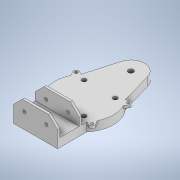
# Autodesk Inventor part: GripperBase
Saved by Autodesk Inventor 2020 (Build 240168000, 168)
## iProperties
Created: 2019-11-04
Part Number: GripperBase
Material: Generic
Document SubType Name: Modeling
Designer: kaspe
Density: 1 g/cm^3
Appearance: Default
Author: kaspe
Autodesk Inventor part; units mm, degrees
ref_plane "YZ Plane" through (0, 0, 0) normal (1, 0, 0) x (0, 1, 0)
ref_plane "XZ Plane" through (0, 0, 0) normal (0, 1, 0) x (-1, 0, 0)
ref_plane "XY Plane" through (0, 0, 0) normal (0, 0, 1) x (1, 0, 0)
sketch "Sketch1" plane through (0, 0, 0) normal (0, 1, 0) x (-1, 0, 0)
  circle A0 centre (0, 0) radius 31.65
  circle A1 centre (0, 0) radius 33.15
  dimension "d0" = 63.3
  dimension "d1" = 66.3
  constraints: 2 centre point, 2 coincident
  measures "d0" diameter of A0
  measures "d1" diameter of A1
extrude "Extrusion1" add sketch "Sketch1" along normal blind 9.8 contours A0 | A1
sketch "Sketch2" plane through (0, 0, 0) normal (0, -1, 0) x (1, 0, 0)
  circle A0 centre (0, 0) radius 31.65
  dimension "d4" = 63.3
  constraints: 1 centre point, 1 coincident
  measures "d4" diameter of A0
extrude "Extrusion2" cut sketch "Sketch2" against normal blind 6.5
sketch "Sketch3" plane through (0, 9.8, 0) normal (0, 1, 0) x (1, 0, 0)
  circle A0 centre (0, 0) radius 25
  line L0 (0, 0) -> (17.6777, 17.6777)
  line L1 (0, 0) -> (25, 0) construction
  line L2 (0, 0) -> (-17.6777, 17.6777)
  line L3 (0, 0) -> (-17.6777, -17.6777)
  line L4 (0, 0) -> (17.6777, -17.6777)
  circle A1 centre (-17.6777, 17.6777) radius 2.55
  circle A2 centre (17.6777, 17.6777) radius 2.55
  circle A3 centre (17.6777, -17.6777) radius 2.55
  circle A4 centre (-17.6777, -17.6777) radius 2.55
  circle A5 centre (0, 25) radius 3.05
  dimension "d7" = 50
  dimension "d8" = 45
  dimension "d9" = 5.1
  dimension "d10" = 5.1
  dimension "d11" = 5.1
  dimension "d12" = 5.1
  dimension "d13" = 6.1
  constraints: 10 end point, 6 centre point, 6 point on circle, 4 coincident, 1 equal length, 1 horizontal, 1 perpendicular, 1 point on line
  measures "d7" diameter of A0
  measures "d8" angle of L1 L0
  measures "d9" diameter of A1
  measures "d10" diameter of A2
  measures "d11" diameter of A3
  measures "d12" diameter of A4
  measures "d13" diameter of A5
extrude "Extrusion3" cut sketch "Sketch3" against normal blind 6.5 contours A2 L0 A0 | A0 A2 | A3 A0 | A0 L4 A3 | L0 A2 A0 | A0 A3 L4 | A5 A0 | A0 A5 | A1 A0 L2 | L2 A0 A1 | A4 A0 L3 | L3 A0 A4 | A4 A0 | A0 A1
sketch "Sketch4" plane through (0, 9.8, 0) normal (0, 1, 0) x (1, 0, 0)
  circle A0 centre (0, 0) radius 33.15 projected
  line L0 (0, 33.15) -> (0, -33.15)
  constraints: 2 end point, 2 point on circle, 1 vertical
ref_plane "Work Plane1" through (0, 9.8, 33.15) normal (0, 0, 1) x (1, 0, 0)
ref_plane "Work Plane2" through (0, 9.8, -33.15) normal (0, 0, -1) x (-1, 0, 0)
sketch "Sketch5" plane through (0, 9.8, -33.15) normal (0, 0, -1) x (-1, 0, 0)
  line L0 (33.15, 0) -> (-33.15, 0) projected
  line L1 (0, 0) -> (25, 0)
  line L2 (0, 0) -> (-25, 0)
  line L3 (33.15, -9.8) -> (-33.15, -9.8) projected
  line L4 (-25, 0) -> (25, 0)
  line L5 (25, 0) -> (25, -9.8)
  line L6 (25, -9.8) -> (-25, -9.8)
  line L7 (-25, -9.8) -> (-25, 0)
  point P0 (0, -9.8)
  dimension "d16" = 25
  dimension "d17" = 25
  constraints: 12 end point, 3 point on line, 2 parallel, 1 horizontal, 1 midpoint, 1 perpendicular
  measures "d16" distance of L1.start L1.end
  measures "d17" distance of L1.start L2.end
extrude "Extrusion4" add sketch "Sketch5" against normal blind 11.75
sketch "Sketch6" plane through (0, 9.8, 33.15) normal (0, 0, 1) x (1, 0, 0)
  line L0 (-25, 0) -> (25, 0) projected
  line L1 (0, 0) -> (-25, 0)
  line L2 (-25, 0) -> (-25, -9.8) projected
  line L3 (25, -9.8) -> (25, 0) projected
  line L4 (-25, 0) -> (25, 0)
  line L5 (25, 0) -> (25, -9.8)
  line L6 (25, -9.8) -> (-25, -9.8)
  line L7 (-25, -9.8) -> (-25, 0)
  point P0 (0, -9.8)
  dimension "d20" = 25
  dimension "d21" = 50
  constraints: 10 end point, 2 parallel, 1 collinear, 1 horizontal, 1 midpoint, 1 perpendicular
  measures "d20" distance of L1.start L0.start
  measures "d21" distance of L3.start L6.end
extrude "Extrusion5" add sketch "Sketch6" against normal blind 12.25
sketch "Sketch8" plane through (0, 9.8, 33.15) normal (0, 0, 1) x (1, 0, 0)
  line L0 (-25, -9.8) -> (25, -9.8) projected
  line L1 (25, 0) -> (25, -9.8) projected
  line L2 (-25, -9.8) -> (25, -9.8)
  line L3 (25, -9.8) -> (25, 0)
  line L4 (25, 0) -> (-25, 0)
  line L5 (-25, 0) -> (-25, -9.8)
  point P0 (0, -9.8)
  constraints: 8 end point, 2 parallel, 1 horizontal, 1 perpendicular
extrude "Extrusion6" add sketch "Sketch8" along normal blind 22
sketch "Sketch9" plane through (0, 9.8, 0) normal (0, 1, 0) x (1, 0, 0)
  line L0 (-25, -55.15) -> (-25, -21.7698) projected
  line L1 (25, -21.7698) -> (25, -55.15) projected
  line L2 (-25, -55.15) -> (25, -55.15)
  line L3 (25, -55.15) -> (25, -52.65)
  line L4 (25, -52.65) -> (-25, -52.65)
  line L5 (-25, -52.65) -> (-25, -55.15)
  point P0 (0, 0)
  dimension "d26" = 2.5
  constraints: 8 end point, 2 parallel, 1 horizontal, 1 perpendicular, 1 point on line
  measures "d26" distance of L3.end L2.end
extrude "Extrusion7" add sketch "Sketch9" along normal blind 19
sketch "Sketch11" plane through (0, 9.8, 0) normal (0, 1, 0) x (1, 0, 0)
  line L0 (25, -21.7698) -> (25, -52.65) projected
  line L1 (-25, -52.65) -> (-25, -21.7698) projected
  line L2 (25, -52.65) -> (-25, -52.65)
  line L3 (-25, -52.65) -> (-25, -30.55)
  line L4 (-25, -30.55) -> (25, -30.55)
  line L5 (25, -30.55) -> (25, -52.65)
  line L6 (25, -30.55) -> (-25, -30.55)
  line L7 (-25, -30.55) -> (-25, -28.05)
  line L8 (-25, -28.05) -> (25, -28.05)
  line L9 (25, -28.05) -> (25, -30.55)
  point P0 (0, 0)
  dimension "d39" = 22.1
  dimension "d40" = 2.5
  constraints: 16 end point, 4 parallel, 2 horizontal, 2 perpendicular, 2 point on line
  measures "d39" distance of L2.end L3.end
  measures "d40" distance of L6.end L7.end
extrude "Extrusion9" add sketch "Sketch11" along normal blind 19 contours L0 L4 L1 L8
sketch "Sketch10" plane through (0, 9.8, 55.15) normal (0, 0, 1) x (1, 0, 0)
  line L0 (-25, 0) -> (25, 0) projected
  line L1 (25, -9.8) -> (25, 19) projected
  line L2 (-25, 0) -> (25, 0)
  line L3 (25, 0) -> (25, 7.8)
  line L4 (25, 7.8) -> (-25, 7.8)
  line L5 (-25, 7.8) -> (-25, 0)
  line L6 (0, 0) -> (12.5, 0)
  line L7 (0, 0) -> (-12.5, 0)
  circle A0 centre (-12.5, 7.8) radius 1.75
  circle A1 centre (12.5, 7.8) radius 1.75
  point P0 (0, -9.8)
  dimension "d29" = 7.8
  dimension "d30" = 12.5
  dimension "d31" = 12.5
  dimension "d32" = 3.5
  dimension "d33" = 3.5
  constraints: 12 end point, 5 point on line, 2 centre point, 2 parallel, 1 horizontal, 1 midpoint, 1 perpendicular
  measures "d29" distance of L3.end L2.end
  measures "d30" distance of L6.start L6.end
  measures "d31" distance of L6.start L7.end
  measures "d32" diameter of A0
  measures "d33" diameter of A1
extrude "Extrusion8" cut sketch "Sketch10" against normal blind 32.5 contours A0 L4 | L4 A0 | A1 L4 | L4 A1
chamfer "Chamfer2" distance 10 angle 45 4 edges at (-25, 28.8, 29.3) (25, 28.8, 29.3) (25, 28.8, 53.9) (-25, 28.8, 53.9)
sketch "Sketch12" plane through (0, 9.8, -33.15) normal (0, 0, -1) x (-1, 0, 0)
  point P0 (0, -9.8)
sketch "Sketch13" plane through (0, 9.8, -33.15) normal (0, 0, -1) x (-1, 0, 0)
  line L0 (-25, 0) -> (-33.15, 0) projected
  line L1 (25, -9.8) -> (-25, -9.8) projected
  line L2 (-25, 0) -> (25, 0)
  line L3 (25, 0) -> (25, -9.8)
  line L4 (25, -9.8) -> (-25, -9.8)
  line L5 (-25, -9.8) -> (-25, 0)
  point P0 (0, -9.8)
  constraints: 8 end point, 2 parallel, 1 horizontal, 1 perpendicular
extrude "Extrusion10" add sketch "Sketch13" along normal blind 35.5
sketch "Sketch14" plane through (0, 9.8, 0) normal (0, 1, 0) x (1, 0, 0)
  line L0 (25, 68.65) -> (-25, 68.65) projected
  line L1 (0, 68.65) -> (0, 53.15)
  circle A0 centre (0, 53.15) radius 3
  point P0 (0, 0)
  dimension "d48" = 15.5
  dimension "d49" = 6
  constraints: 2 end point, 1 centre point, 1 coincident, 1 midpoint, 1 vertical
  measures "d48" distance of L1.start L1.end
  measures "d49" diameter of A0
extrude "Extrusion11" cut sketch "Sketch14" against normal blind 32.5
sketch "Sketch15" plane through (0, 9.8, 0) normal (0, 1, 0) x (1, 0, 0)
  circle A0 centre (0, 53.15) radius 3 projected
  circle A1 centre (0, 53.15) radius 15.5
  line L0 (25, 21.7698) -> (25, 68.65) projected
  line L1 (25, 21.7698) -> (14.9131, 57.3749)
  line L2 (-25, 68.65) -> (-25, 21.7698) projected
  line L3 (-25, 21.7698) -> (-14.9131, 57.3749)
  arc A2 (25, -21.7698) -> (25, 21.7698) centre (0, 0) ccw projected
  arc A3 (-25, 21.7698) -> (-25, -21.7698) centre (0, 0) ccw projected
  arc A4 (25, 21.7698) -> (-25, 21.7698) centre (0, 0) ccw
  line L4 (25, 68.65) -> (-25, 68.65)
  line L5 (-25, 68.65) -> (-25, 21.7698)
  line L6 (-25, 21.7698) -> (25, 21.7698)
  line L7 (25, 21.7698) -> (25, 68.65)
  point P0 (0, 68.65)
  dimension "d52" = 31
  constraints: 12 end point, 4 point on circle, 2 centre point, 2 parallel, 2 tangent, 1 coincident, 1 horizontal, 1 perpendicular
  measures "d52" diameter of A1
extrude "Extrusion12" cut sketch "Sketch15" against normal blind 32.5 contours A1 L4 L0 L1 | L3 L2 L4 A1
sketch "Sketch16" plane through (0, 9.8, 0) normal (0, 1, 0) x (1, 0, 0)
  arc A0 (25, -21.7698) -> (25, 21.7698) centre (0, 0) ccw projected
  line L0 (0, 0) -> (33.15, 0) construction
  line L1 (0, 0) -> (33.15, 0) construction
  arc A1 (-25, 21.7698) -> (-25, -21.7698) centre (0, 0) ccw projected
  circle A2 centre (29.6581, -20.6675) radius 1.65
  circle A3 centre (29.6123, 20.7348) radius 1.65
  circle A4 centre (-29.733, 20.7307) radius 1.65
  circle A5 centre (-29.6123, -20.7348) radius 1.65
  arc A6 (-32.1853, -19.1921) -> (-28.2622, -23.4138) centre (-29.6123, -20.7348) ccw
  arc A7 (-28.424, 23.4301) -> (-32.3413, 19.2486) centre (-29.733, 20.7307) ccw
  line L2 (-29.733, 20.7307) -> (-25.8681, 20.7307)
  line L3 (29.6508, -14.824) -> (32.2307, -19.1241)
  line L4 (29.6187, 14.8881) -> (32.189, 19.1982)
  line L5 (-29.733, 14.6585) -> (-32.3413, 19.2486)
  line L6 (-29.6123, -14.9007) -> (-32.1853, -19.1921)
  line L7 (25, 21.7698) -> (28.2622, 23.4138)
  line L8 (-14.9131, 57.3749) -> (-25, 21.7698) projected
  line L9 (-25, 21.7698) -> (-28.424, 23.4301)
  line L10 (-25, -21.7698) -> (-28.2622, -23.4138)
  line L11 (25, -21.7698) -> (25, -28.05) projected
  line L12 (25, -21.7698) -> (28.3668, -23.3753)
  arc A8 (32.189, 19.1982) -> (28.2622, 23.4138) centre (29.6123, 20.7348) ccw
  arc A9 (27.2402, -18.8916) -> (26.6581, -20.6712) centre (29.6581, -20.6675) ccw
  arc A10 (28.3668, -23.3753) -> (32.2307, -19.1241) centre (29.6581, -20.6675) ccw
  point P0 (25.8681, 20.7307)
  point P1 (25.915, -20.6721)
  point P2 (27.1549, 19.0141)
  point P3 (26.6123, 20.7315)
  point P4 (27.1549, -19.0141)
  dimension "d58" = 3.3
  dimension "d62" = 3.3
  dimension "d63" = 3.3
  constraints: 22 end point, 19 point on circle, 9 centre point, 8 tangent, 4 coincident, 2 horizontal, 1 point on line
  measures "d58" diameter of A2
  measures "d62" diameter of A3
  measures "d63" diameter of A4
extrude "Extrusion13" add sketch "Sketch16" against normal blind 3
body "Solid1"
